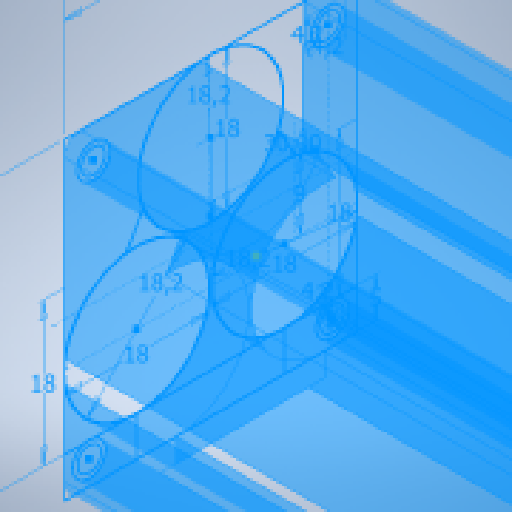
# Autodesk Inventor part: akkum_wall
Saved by Autodesk Inventor 2023 (Build 270158000, 158)
## iProperties
Created: 2026-02-15
Part Number: akkum_wall
Material: Типовые
Document SubType Name: Modeling
Designer: garin
Density: 1 g/cm^3
Appearance: По умолчанию
Author: garin
Autodesk Inventor part; units mm, degrees
ref_plane "YZ Plane" through (0, 0, 0) normal (1, 0, 0) x (0, 1, 0)
ref_plane "XZ Plane" through (0, 0, 0) normal (0, 1, 0) x (-1, 0, 0)
ref_plane "XY Plane" through (0, 0, 0) normal (0, 0, 1) x (1, 0, 0)
sketch "Эскиз1" plane through (0, 0, 0) normal (0, 0, 1) x (1, 0, 0)
  line L0 (0, 0) -> (6.3273, 0) construction
  line L1 (6.3273, 0) -> (6.3273, -4.5) construction
  line L2 (6.3273, -4.5) -> (0, -4.5) construction
  line L3 (0, -4.5) -> (0, 0) construction
  line L4 (6.3273, -4.5) -> (-32.7727, -4.5)
  line L5 (-32.7727, -4.5) -> (-32.7727, 32)
  line L6 (-32.7727, 32) -> (6.3273, 32)
  line L7 (6.3273, 32) -> (6.3273, -4.5)
  line L8 (6.3273, 13.75) -> (-32.7727, 13.75) construction
  line L9 (-13.2227, -4.5) -> (-13.2227, 32) construction
  line L10 (6.3273, -4.5) -> (3.3273, -4.5) construction
  line L11 (6.3273, -1.45) -> (6.3273, -4.5) construction
  circle A0 centre (3.3273, 28.95) radius 1.5
  circle A1 centre (3.3273, -1.45) radius 1.5
  line L12 (-32.7727, -4.5) -> (-28.6727, -4.5)
  circle A2 centre (-28.6727, -0.9) radius 1.5
  circle A3 centre (-28.6727, 28.4) radius 1.5
  line L13 (-32.7727, -4.5) -> (-32.7727, 2.1)
  line L14 (-32.7727, 2.1) -> (0, 2.1)
  line L15 (0, 2.1) -> (0, 25.4)
  line L16 (0, 25.4) -> (-32.7727, 25.4)
  line L17 (-32.7727, 25.4) -> (-32.7727, 2.1)
  line L18 (0, 13.75) -> (0, 21.25) construction
  line L19 (0, 21.25) -> (-32.7727, 21.25)
  line L20 (-32.7727, 21.25) -> (-32.7727, 6.25)
  line L21 (-32.7727, 6.25) -> (0, 6.25)
  line L22 (0, 6.25) -> (0, 21.25)
  line L23 (-32.7727, 21.25) -> (-34.7727, 21.25)
  line L24 (-34.7727, 21.25) -> (-34.7727, 6.25)
  line L25 (-34.7727, 6.25) -> (-32.7727, 6.25)
  line L26 (-32.7727, 6.25) -> (-32.7727, 21.25)
  line L27 (-32.7727, 6.25) -> (-25.2727, 6.25)
  line L28 (-25.2727, 6.25) -> (-25.2727, 21.25)
  line L29 (-25.2727, 21.25) -> (-32.7727, 21.25)
  line L30 (-32.7727, 21.25) -> (-32.7727, 6.25)
  line L31 (-32.7727, 6.25) -> (0, 6.25)
  line L32 (0, 6.25) -> (0, 5.25)
  line L33 (0, 5.25) -> (-32.7727, 5.25)
  line L34 (-32.7727, 5.25) -> (-32.7727, 6.25)
  line L35 (0, 21.25) -> (-32.7727, 21.25)
  line L36 (-32.7727, 21.25) -> (-32.7727, 22.25)
  line L37 (-32.7727, 22.25) -> (0, 22.25)
  line L38 (0, 22.25) -> (0, 21.25)
  line L39 (-32.7727, 13.75) -> (-22.4946, 25.4)
  line L40 (-32.7727, 13.75) -> (-17.2369, 13.75) construction
  line L41 (-32.7727, 13.75) -> (-22.4946, 2.1)
  dimension "d0" = 39.1
  dimension "d1" = 36.5
  dimension "d8" = 3
  dimension "d9" = 3
  dimension "d11" = 3
  dimension "d12" = 3
  dimension "d13" = 6.6
  dimension "d19" = 7.5
  dimension "d20" = 15
  dimension "d21" = 2
  dimension "d22" = 7.5
  dimension "d23" = 1
  dimension "d24" = 1
  dimension "d35" = 48.58
  constraints: 84 end point, 16 parallel, 11 horizontal, 8 perpendicular, 8 point on line, 6 coincident, 5 midpoint, 4 centre point, 4 symmetric about line, 1 equal length
  measures "d0" distance of L5.end L6.end
  measures "d1" distance of L4.end L5.end
  measures "d8" diameter of A0
  measures "d9" diameter of A1
  measures "d11" diameter of A2
  measures "d12" diameter of A3
  measures "d13" distance of L4.end L13.end
  measures "d19" distance of L18.start L18.end
  measures "d20" distance of L20.end L19.end
  measures "d21" distance of L25.end L24.end
  measures "d22" distance of L29.end L28.end
  measures "d23" distance of L31.end L32.end
  measures "d24" distance of L35.end L36.end
  measures "d35" angle of L40 L39
extrude "Выдавливание1" add sketch "Эскиз1" along normal blind 5 contours L4 L5 L14 L15 L16 L6 L7 | L5 L33 L41 L14 | L16 L39 L37 L5 | L5 L21 L41 L33 | L41 L33 L15 L14 | L37 L39 L19 L5 | L16 L15 L37 L39 | L5 L41 L21 | L41 L21 L15 L33 | L19 L39 L5 | L37 L15 L19 L39 | L39 L19 L28 L21 L41 | L28 L19 L15 L21
extrude "Выдавливание2" cut sketch "Эскиз1" along normal blind 2 contours L5 L33 L41 L14 | L16 L39 L37 L5 | L5 L21 L41 L33 | L41 L33 L15 L14 | L37 L39 L19 L5 | L16 L15 L37 L39 | L5 L41 L21 | L41 L21 L15 L33 | L19 L39 L5 | L37 L15 L19 L39 | L39 L19 L28 L21 L41 | L28 L19 L15 L21
fillet "Сопряжение1" radius 2 4 edges at (-32.7727, -4.5, 2.5) (6.3273, -4.5, 2.5) (6.3273, 32, 2.5) (-32.7727, 32, 2.5)
extrude "Выдавливание3" cut sketch "Эскиз1" along normal blind 5 contours L5 L21 L41 L33 | L37 L39 L19 L5 | L41 L21 L15 L33 | L37 L15 L19 L39
extrude "Выдавливание4" add sketch "Эскиз1" along normal blind 3 from surface at 2 contours L25 L24 L23 L5
extrude "Выдавливание5" cut sketch "Эскиз1" against normal blind 1.5 from surface at 5 contours L5 L41 L21 | L19 L39 L5 | L39 L19 L28 L21 L41
fillet "Сопряжение2" radius 2 1 edges at (-32.7727, 13.75, 3.5)
chamfer "Фаска1" distance 1.5 angle 45 4 edges at (-30.1727, 28.4, 5) (-30.1727, -0.9, 5) (1.8273, -1.45, 5) (1.8273, 28.95, 5)
extrude "Выдавливание6" add sketch "Эскиз1" along normal blind 1.5 contours L5 L33 L41 L14 | L16 L39 L37 L5 | L5 L21 L41 L33 | L37 L39 L19 L5 | L5 L41 L21 | L19 L39 L5
